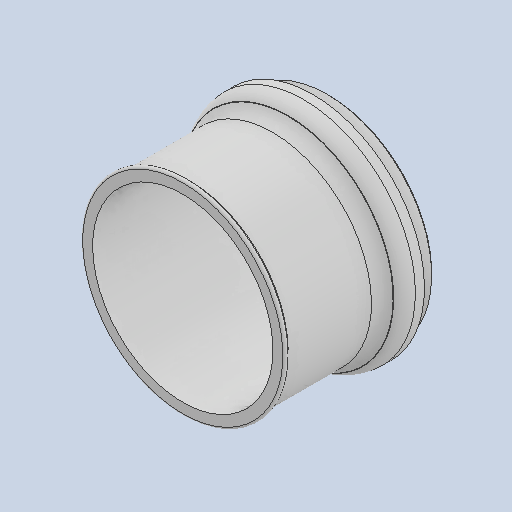
# Autodesk Inventor part: servoCushionSleeve
Saved by Autodesk Inventor 2023 (Build 270158000, 158)
## iProperties
Created: 2023-06-25
Part Number: servoCushionSleeve
Material: Типовые
Document SubType Name: Modeling
Designer: khrip
Density: 1 g/cm^3
Appearance: По умолчанию
Author: khrip
Autodesk Inventor part; units mm, degrees
ref_plane "YZ Plane" through (0, 0, 0) normal (1, 0, 0) x (0, 1, 0)
ref_plane "XZ Plane" through (0, 0, 0) normal (0, 1, 0) x (-1, 0, 0)
ref_plane "XY Plane" through (0, 0, 0) normal (0, 0, 1) x (1, 0, 0)
sketch "Эскиз1" plane through (0, 0, 0) normal (1, 0, 0) x (0, 1, 0)
  line L0 (-13.5, 0) -> (13.5, 0)
  line L1 (-14.5, 0) -> (13.5, 0)
  line L2 (-13.5, -2.3) -> (13.5, -2.3) projected
  line L3 (12.5, 18) -> (12.5, 1)
  line L4 (12.5, 1) -> (12.5, 0)
  line L5 (12.5, 0) -> (12.5, 18)
  line L6 (12.5, 0) -> (13.5, 0)
  line L7 (13.5, 0) -> (13.5, -2.3)
  line L8 (13.5, -2.3) -> (14.5, -2.3)
  line L9 (14.5, -2.3) -> (14.5, 0)
  line L10 (15.5, 0) -> (15.5, -3.3)
  line L11 (14.5, 0) -> (15.5, 0)
  line L12 (15.5, 0) -> (15.5, 2.5)
  line L13 (12.5, 18) -> (13.7, 18)
  line L14 (13.7, 17.1) -> (13.7, 4.3)
  line L15 (14.5, 2.5) -> (15.5, 2.5)
  line L16 (15.5, 2.5) -> (13.7, 4.3)
  line L17 (15.5, 2.5) -> (19.4703, 2.5) construction
  line L18 (13.7, 18) -> (14.6, 18)
  line L19 (14.6, 18) -> (13.7, 17.1)
  line L20 (0, -7.56) -> (0, 22.26) projected
  point P0 (0, 0)
  point P1 (12.5, 0)
  dimension "d0" = 18
  dimension "d1" = 2.5
  dimension "d2" = 1.2
  dimension "d3" = 135
  dimension "d4" = 45
  constraints: 38 end point, 5 horizontal, 4 perpendicular, 4 point on line, 3 vertical, 1 collinear, 4 other
  measures "d0" distance of L4.end L5.end
  measures "d1" distance of L10.start L12.end
  measures "d2" distance of L5.end L13.end
  measures "d3" angle of L17 L16
  measures "d4" angle of L18 L19
revolve "Вращение1" add sketch "Эскиз1" angle 360 about axis through (0, 0, -10) along (0, 0, 1) contours L4 L3 L13 L18 L19 L14 L16 L12 L11 L9 L8 L7 L0
chamfer "Фаска1" distance 0.3 angle 45 2 edges at (0, -14.5, -2.3) (0, -13.5, -2.3)
fillet "Сопряжение1" radius 0.3 1 edges at (0, -14.6, 18)
fillet "Сопряжение2" radius 3 2 edges at (0, -13.7, 4.3) (0, -15.5, 2.5)
